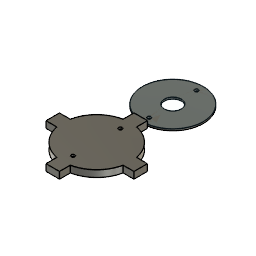
Stage 2 (Autodesk Fusion 360 design; units mm, degrees)
part number: 2025-11-29-20-59-17-478
Autodesk Fusion 360 part; units mm, degrees
note: some values were not read from the file. Chosen so that the rebuilt part matches the saved one: that a step has no effect.
sketch "Sketch1" plane through (0, 0, 0) normal (0, 0, 1) x (1, 0, 0)
sketch "Sketch2" plane through (0, 0, 0) normal (0, 0, 1) x (1, 0, 0)
  circle A0 centre (0, 0) radius 100
  constraint coincident A0.centre origin
extrude "Extrude1" add sketch "Sketch2" along normal blind 70 makes body 1
sketch "Sketch3" plane through (0, 0, 0) normal (0, 0, 1) x (1, 0, 0)
  circle A0 centre (0, -70) radius 17.5
  circle A1 centre (0, 70) radius 17.5
  dimension "d3" = 35
  dimension "d4" = 35
  measures "d3" diameter of A0
  measures "d4" diameter of A1
extrude "Extrude2" cut sketch "Sketch3" along normal blind 15 bodies 1
sketch "Sketch4" plane through (0, 0, 0) normal (0, 0, 1) x (1, 0, 0)
  circle A0 centre (0, -70) radius 5.25
  circle A1 centre (0, 70) radius 5.25
  dimension "d7" = 10.5
  dimension "d8" = 10.5
  measures "d7" diameter of A0
  measures "d8" diameter of A1
extrude "Extrude3" cut sketch "Sketch4" along normal blind 90 bodies 1
extrude "Extrude4" cut 1 faces at (34.612, 0, 70) along direction (0, 0, -1) blind 20 on bodies 1 bodies 1
extrude "Extrude5" cut 1 faces at (34.612, 0, 50) along direction (0, 0, -1) blind 20 on bodies 1 bodies 1
sketch "Sketch5" plane through (0, 0, 30) normal (0, 0, 1) x (-1, 0, 0)
  circle A0 centre (0, -70) radius 5.25
  circle A1 centre (0, 70) radius 5.25
  circle A2 centre (0, 0) radius 100
  circle A3 centre (0, 0) radius 50
  constraint coincident A2.centre A3.centre
extrude "Extrude6" cut sketch "Sketch5" against normal blind 15 contours A3 bodies 1
sketch "Sketch6" plane through (0, 0, 0) normal (0, 0, 1) x (1, 0, 0)
  line L0 (125, -10) -> (90, -10)
  line L1 (90, -10) -> (90, 15)
  line L2 (90, 15) -> (125, 15)
  line L3 (125, 15) -> (125, -10)
  constraint horizontal L0
  constraint vertical L1
  constraint horizontal L2
  constraint vertical L3
extrude "Extrude7" add sketch "Sketch6" along normal blind 10 separate body makes body 2
move_body "Move1" bodies 2 to x (1, 0, 0) y (0, 1, 0) z (0, 0, 1) at (0, -2.5, 0)
sketch "Sketch7" plane through (0, 0, 15) normal (0, 0, 1) x (-1, 0, 0)
  circle A0 centre (0, 0) radius 50
sketch "Sketch8" plane through (0, 12.5, 0) normal (0, 1, 0) x (-1, 0, 0)
  line L0 (-125, 0) -> (-90, 0)
  line L1 (-90, 0) -> (-90, 10)
  line L2 (-90, 10) -> (-125, 10)
  line L3 (-125, 10) -> (-125, 0)
  line L4 (-125, 0) -> (-100, 10)
  line L5 (-125, 10) -> (-125, 0)
  constraint coincident L0.start L3.end
  constraint coincident L2 L4.end
  constraint coincident L2.end L3.start
combine "Combine1" operation add target body 2 tool bodies 1
combine "Combine2" [no effect]
combine "Combine3" [no effect]
combine "Combine4" [no effect]
combine "Combine5" [no effect]
sketch "Sketch9" plane through (0, 0, 30) normal (0, 0, 1) x (-1, 0, 0)
  circle A0 centre (0, 0) radius 50
  circle A1 centre (0, -70) radius 5.25
  circle A2 centre (0, 70) radius 5.25
  circle A3 centre (0, 0) radius 100
  circle A4 centre (220, -250) radius 90
extrude "Extrude9" add sketch "Sketch9" along normal blind 5 separate body contours A4 makes body 3
sketch "Sketch10" plane through (0, 0, 30) normal (0, 0, 1) x (-1, 0, 0)
  circle A0 centre (0, 0) radius 50
  circle A1 centre (0, -70) radius 5.25
  circle A2 centre (0, 70) radius 5.25
  circle A3 centre (0, 0) radius 100
sketch "Sketch11" plane through (0, 0, 35) normal (0, 0, 1) x (-1, 0, 0)
  circle A0 centre (220, -250) radius 90
  circle A1 centre (290, -250) radius 5.25
  circle A2 centre (150, -250) radius 5.25
  dimension "d23" = 10.5
  dimension "d24" = 10.5
  measures "d23" diameter of A1
  measures "d24" diameter of A2
extrude "Extrude10" cut sketch "Sketch11" against normal blind 40 contours A1 | A2 bodies 3
move_body "Move5" bodies 3 to x (1, 0, 0) y (0, 1, 0) z (0, 0, 1) at (0, 0, -30)
sketch "Sketch12" plane through (0, 0, 30) normal (0, 0, 1) x (-1, 0, 0)
  circle A0 centre (220, -250) radius 25
  dimension "d27" = 50
  measures "d27" diameter of A0
extrude "Extrude11" cut sketch "Sketch12" against normal blind 30 bodies 3
sketch "Sketch13" plane through (0, 0, 0) normal (0, 0, 1) x (1, 0, 0)
extrude "Extrude12" cut sketch "Sketch10" against normal blind 10 bodies 2
move_body "Move6" bodies 3 to x (0, -1, 0) y (1, 0, 0) z (0, 0, 1) at (-495, 5, 0)
move_body "Move7" bodies 3 to x (1, 0, 0) y (0, 1, 0) z (0, 0, 1) at (240, 0, 0)
move_body "Move8" bodies 3 to x (1, 0, 0) y (0, 1, 0) z (0, 0, 1) at (5, 0, 0)
sketch "Sketch14" plane through (0, 0, 5) normal (0, 0, 1) x (-1, 0, 0)
  circle A0 centre (0, -225) radius 25
  circle A1 centre (0, -295) radius 5.25
  circle A2 centre (0, -155) radius 5.25
  circle A3 centre (0, -225) radius 90
extrude "Extrude13" cut 1 faces at (116.6667, 0, 10) along direction (0, 0, -1) blind 30 on bodies 2 bodies 2
sketch "Sketch15" plane through (0, 0, 0) normal (0, 0, 1) x (1, 0, 0)
  circle A0 centre (0, 0) radius 50
  constraint coincident A0.centre origin
extrude "Extrude14" cut sketch "Sketch15" along normal blind 10 bodies 2
extrude "Extrude15" add sketch "Sketch7" along normal blind 5 bodies 2
extrude "Extrude16" cut 1 faces at (-13.5518, -2.484, 10) along direction (0, 0, 1) blind 5 on bodies 2 bodies 2
sketch "Sketch16" plane through (0, 0, 20) normal (0, 0, 1) x (-1, 0, 0)
  circle A0 centre (0, 70) radius 5.25
  circle A1 centre (0, -70) radius 5.25
  circle A2 centre (0, 0) radius 100
  line L0 (-20, -120) -> (20, -120)
  line L1 (20, -120) -> (20, -90)
  line L2 (20, -90) -> (-20, -90)
  line L3 (-20, -90) -> (-20, -120)
  constraint horizontal L0
  constraint perpendicular L0 L1
  constraint perpendicular L1 L2
  constraint perpendicular L0 L3
extrude "Extrude17" add sketch "Sketch16" against normal blind 20 contours A2 L0 L1 L3 bodies 2
sketch "Sketch17" plane through (0, 0, 20) normal (0, 0, 1) x (-1, 0, 0)
  circle A0 centre (0, 70) radius 5.25
  circle A1 centre (0, -70) radius 5.25
  arc A2 (20, -97.9796) -> (-20, -97.9796) centre (0, 0) ccw
  line L0 (-20, -97.9796) -> (-20, -120)
  line L1 (-20, -120) -> (20, -120)
  line L2 (20, -120) -> (20, -97.9796)
  line L3 (-20, 90) -> (20, 90)
  line L4 (20, 90) -> (20, 120)
  line L5 (20, 120) -> (-20, 120)
  line L6 (-20, 120) -> (-20, 90)
  line L7 (-90, 20) -> (-120, 20)
  line L8 (-120, 20) -> (-120, -20)
  line L9 (-120, -20) -> (-90, -20)
  line L10 (-90, -20) -> (-90, 20)
  line L11 (120, -20) -> (90, -20)
  line L12 (90, -20) -> (90, 20)
  line L13 (90, 20) -> (120, 20)
  line L14 (120, 20) -> (120, -20)
  constraint horizontal L3
  constraint vertical L4
  constraint horizontal L5
  constraint vertical L6
  constraint horizontal L7
  constraint vertical L8
  constraint horizontal L9
  constraint vertical L10
  constraint horizontal L11
  constraint vertical L12
  constraint horizontal L13
  constraint vertical L14
extrude "Extrude18" add sketch "Sketch17" against normal blind 20 contours A2 L11 L13 L14 | A2 L4 L5 L6 | A2 L7 L8 L9 bodies 2
extrude "Extrude19" add 1 faces at (-120, -6.6667, 13.3333) along direction (-1, 0, 0) blind 10 on bodies 2 bodies 2
extrude "Extrude20" add 1 faces at (-6.6667, -120, 13.3333) along direction (0, -1, 0) blind 10 on bodies 2 bodies 2
extrude "Extrude21" add 1 faces at (120, -6.6667, 13.3333) along direction (1, 0, 0) blind 10 on bodies 2 bodies 2
extrude "Extrude22" add 1 faces at (6.6667, 120, 13.3333) along direction (0, 1, 0) blind 10 on bodies 2 bodies 2
